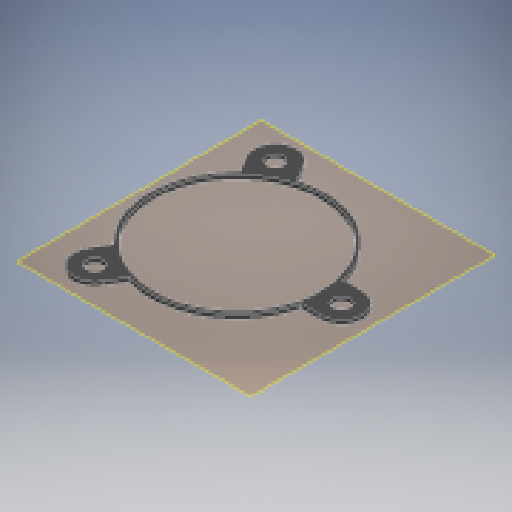
# Autodesk Inventor part: CE-8.2.1-01-001
Saved by Autodesk Inventor 2024 (Build 280153000, 153)
## iProperties
Created: 2024-03-07
Part Number: CE-8.2.1-01-001
Material: Rubber
Document SubType Name: Modeling
Designer: Alex
Density: 0.93 g/cm^3
Appearance: Rubber - Black
Author: Alex
Autodesk Inventor part; units mm, degrees
ref_plane "YZ Plane" through (0, 0, 0) normal (1, 0, 0) x (0, 1, 0)
ref_plane "XZ Plane" through (0, 0, 0) normal (0, 1, 0) x (-1, 0, 0)
ref_plane "XY Plane" through (0, 0, 0) normal (0, 0, 1) x (1, 0, 0)
ref_plane "Work Plane1" through (24.8871, -5.6967, -26.1904) normal (0, 1, 0) x (-1, 0, 0)
sketch "Sketch1" plane through (24.8871, -5.6967, -26.1904) normal (0, 1, 0) x (-1, 0, 0)
  circle A0 centre (12.5, 21.6506) radius 2 projected
  circle A1 centre (12.5, -21.6506) radius 2 projected
  circle A2 centre (-25, 0) radius 2 projected
  arc A3 (-20.3961, -5) -> (5.8679, -20.1635) centre (0, 0) ccw projected
  line L0 (8.1699, -24.1506) -> (5.8679, -20.1635) projected
  arc A4 (8.1699, -24.1506) -> (16.8301, -19.1506) centre (12.5, -21.6506) ccw projected
  line L1 (14.5282, -15.1635) -> (16.8301, -19.1506) projected
  arc A5 (14.5282, -15.1635) -> (14.5282, 15.1635) centre (0, 0) ccw projected
  line L2 (16.8301, 19.1506) -> (14.5282, 15.1635) projected
  arc A6 (16.8301, 19.1506) -> (8.1699, 24.1506) centre (12.5, 21.6506) ccw projected
  line L3 (5.8679, 20.1635) -> (8.1699, 24.1506) projected
  arc A7 (5.8679, 20.1635) -> (-20.3961, 5) centre (0, 0) ccw projected
  line L4 (-25, 5) -> (-20.3961, 5) projected
  arc A8 (-25, 5) -> (-25, -5) centre (-25, 0) ccw projected
  line L5 (-20.3961, -5) -> (-25, -5) projected
  circle A9 centre (0, 0) radius 20 projected
  point P0 (24.8871, 26.1904)
extrude "Extrusion1" add sketch "Sketch1" along normal blind 1
body "Solid1"
